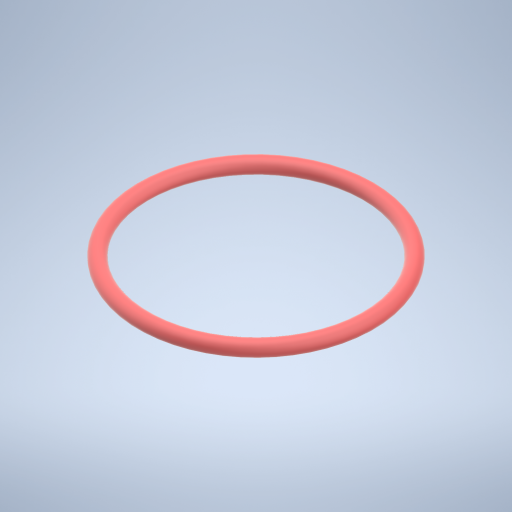
# Autodesk Inventor part: RING
Saved by Autodesk Inventor 2023 (Build 270158000, 158)
## iProperties
Created: 2022-09-29
Part Number: RING
Material: ゴム、シリコーン
Document SubType Name: Modeling
Designer: zegi
Density: 1.25 g/cm^3
Appearance: 滑らか - 赤
Author: zegi
Autodesk Inventor part; units mm, degrees
ref_plane "YZ Plane" through (0, 0, 0) normal (1, 0, 0) x (0, 1, 0)
ref_plane "XZ Plane" through (0, 0, 0) normal (0, 1, 0) x (-1, 0, 0)
ref_plane "XY Plane" through (0, 0, 0) normal (0, 0, 1) x (1, 0, 0)
sketch "スケッチ1" plane through (0, 0, 0) normal (0, 0, 1) x (1, 0, 0)
  circle A0 centre (-107, 0) radius 7
  line L0 (0, 0) -> (0, 50)
  point P0 (-114, 0)
  dimension "d2" = 14
  dimension "d0" = 0
  dimension "d1" = 107
  dimension "d3" = 50
  dimension "d5" = 114
  constraints: 2 end point, 1 coincident, 1 horizontal alignment, 1 vertical, 2 other
  measures "d0" vertical distance of L0.start point (-107, 0)
  measures "d1" distance of point (-107, 0) L0.start
  measures "d3" distance of L0.start L0.end
  measures "d5" distance of L0.start point (-114, 0)
revolve "回転1" add sketch "スケッチ1" angle 360 about axis through (0, 0, 0) along (0, 1, 0)
